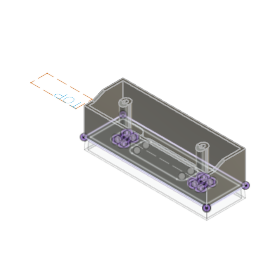
Eufy Doorbell Spacer (Autodesk Fusion 360 design; units mm, degrees)
Autodesk Fusion 360 part; units mm, degrees
note: some values were not read from the file. Chosen so that the rebuilt part matches the saved one: which pieces of a blend or face edit are solid.
sketch "Sketch1" plane through (0, 0, 0) normal (0, 0, 1) x (1, 0, 0) in component "Doorbell Back"
  line L0 (0, 0) -> (147, 0)
  line L1 (147, 0) -> (147, 45.8)
  line L2 (147, 45.8) -> (0, 45.8)
  line L3 (0, 45.8) -> (0, 0)
  line L4 (145.7948, 3.1933) -> (145.7948, 0) construction
  line L5 (145.7948, 43.4933) -> (145.7948, 45.8) construction
  line L6 (147, 22.9) -> (0, 22.9) construction
  line L7 (27.9, 21.95) -> (27.9, 23.85)
  arc A0 (27.9, 23.85) -> (23.8, 23.85) centre (25.85, 23.85) ccw
  line L8 (23.8, 23.85) -> (23.8, 21.95)
  arc A1 (23.8, 21.95) -> (27.9, 21.95) centre (25.85, 21.95) ccw
  line L9 (25.85, 21.95) -> (25.85, 23.85) construction
  line L10 (121, 21.95) -> (121, 23.85)
  arc A2 (121, 23.85) -> (116.9, 23.85) centre (118.95, 23.85) ccw
  line L11 (116.9, 23.85) -> (116.9, 21.95)
  arc A3 (116.9, 21.95) -> (121, 21.95) centre (118.95, 21.95) ccw
  line L12 (118.95, 21.95) -> (118.95, 23.85) construction
  line L13 (22.4, 31.3) -> (29.3, 31.3)
  line L14 (32.3, 28.3) -> (32.3, 17.5)
  line L15 (29.3, 14.5) -> (22.4, 14.5)
  line L16 (19.4, 17.5) -> (19.4, 28.3)
  line L17 (19.4, 31.3) -> (32.3, 14.5) construction
  line L18 (32.3, 31.3) -> (19.4, 14.5) construction
  arc A4 (19.4, 17.5) -> (22.4, 14.5) centre (22.4, 17.5) ccw
  arc A5 (29.3, 14.5) -> (32.3, 17.5) centre (29.3, 17.5) ccw
  arc A6 (22.4, 31.3) -> (19.4, 28.3) centre (22.4, 28.3) ccw
  arc A7 (32.3, 28.3) -> (29.3, 31.3) centre (29.3, 28.3) ccw
  line L19 (25.85, 22.9) -> (118.95, 22.9) construction
  line L20 (115.5, 31.3) -> (122.4, 31.3)
  line L21 (125.4, 28.3) -> (125.4, 17.5)
  line L22 (122.4, 14.5) -> (115.5, 14.5)
  line L23 (112.5, 17.5) -> (112.5, 28.3)
  line L24 (112.5, 31.3) -> (125.4, 14.5) construction
  line L25 (125.4, 31.3) -> (112.5, 14.5) construction
  arc A8 (115.5, 31.3) -> (112.5, 28.3) centre (115.5, 28.3) ccw
  arc A9 (125.4, 28.3) -> (122.4, 31.3) centre (122.4, 28.3) ccw
  arc A10 (122.4, 14.5) -> (125.4, 17.5) centre (122.4, 17.5) ccw
  arc A11 (112.5, 17.5) -> (115.5, 14.5) centre (115.5, 17.5) ccw
  point P0 (25.85, 22.9)
  point P1 (118.95, 22.9)
  point P2 (25.85, 22.9)
  point P3 (118.95, 22.9)
  dimension "d1" = 45.8
  dimension "d5" = 147
  dimension "d6" = 4.1
  dimension "d7" = 6
  dimension "d10" = 16.8
  dimension "d11" = 12.9
  dimension "d12" = 3
  dimension "d14" = 93.1
  dimension "d15" = 28.05
  constraint horizontal L0
  constraint vertical L1
  constraint horizontal L2
  constraint vertical L3
  constraint coincident L0.start L3.end
  constraint coincident L0 L4.end
  constraint perpendicular L0 L4
  constraint coincident L2 L5.end
  constraint perpendicular L2 L5
  constraint midpoint L1 L6.start
  constraint midpoint L3 L6.end
  constraint tangent L7 A0
  constraint tangent A0 L8
  constraint parallel L7 L8
  constraint tangent L8 A1
  constraint tangent L7 A1
  constraint perpendicular L6 L9
  constraint coincident L6 P2
  constraint midpoint L9 P2
  constraint tangent L10 A2
  constraint tangent A2 L11
  constraint parallel L10 L11
  constraint tangent L11 A3
  constraint tangent L10 A3
  constraint perpendicular L6 L12
  constraint midpoint L12 P3
  constraint equal L7 L11
  constraint equal A0 A2
  constraint coincident L6 P3
  constraint horizontal L13
  constraint perpendicular L13 L14
  constraint parallel L13 L15
  constraint parallel L14 L16
  constraint coincident L17 P2
  constraint coincident L18 P2
  constraint coincident P2 P0
  constraint coincident L18.end L15
  constraint coincident L18.end L16
  constraint tangent L15 A4
  constraint tangent L16 A4
  constraint coincident L17.end L14
  constraint coincident L17.end L15
  constraint tangent L14 A5
  constraint tangent L15 A5
  constraint equal A4 A5
  constraint coincident L17.start L16
  constraint coincident L17.start L13
  constraint tangent L16 A6
  constraint tangent L13 A6
  constraint coincident L18.start L14
  constraint coincident L18.start L13
  constraint tangent L14 A7
  constraint tangent L13 A7
  constraint equal A6 A7
  constraint equal A4 A6
  constraint coincident P3 P1
  constraint horizontal L20
  constraint perpendicular L20 L21
  constraint parallel L20 L22
  constraint parallel L21 L23
  constraint coincident L24 P3
  constraint coincident L25 P3
  constraint coincident L24.start L23
  constraint coincident L24.start L20
  constraint tangent L23 A8
  constraint tangent L20 A8
  constraint coincident L25.start L21
  constraint coincident L25.start L20
  constraint tangent L21 A9
  constraint tangent L20 A9
  constraint equal A8 A9
  constraint coincident L24.end L21
  constraint coincident L24.end L22
  constraint tangent L21 A10
  constraint tangent L22 A10
  constraint equal A8 A10
  constraint coincident L25.end L22
  constraint coincident L25.end L23
  constraint tangent L22 A11
  constraint tangent L23 A11
  constraint equal L13 L20
  constraint equal L16 L23
  constraint equal A10 A11
  constraint equal A5 A11
  measures "d1" distance of L0.end L1.end
  measures "d5" distance of L0.start L0.end
  measures "d6" distance of L10 L11
  measures "d10" distance of L18.start L17.end
  measures "d11" distance of L17.end L18.end
  measures "d12" radius of A4
  measures "d14" distance of P2 P3
  measures "d15" distance of L1 P3
extrude "Extrude1" add sketch "Sketch1" against normal blind 13.45 draft 3 contours L0 L1 L2 L3 | L13 L14 L15 L16 A4 A5 A6 A7 | L20 L21 L22 L23 A8 A9 A10 A11 makes body 1 in component "Doorbell Back"
extrude "Extrude2" add sketch "Sketch1" along normal blind 2.8 contours L13 L14 L15 L16 A4 A5 A6 A7 | L20 L21 L22 L23 A8 A9 A10 A11 bodies 1 in component "Doorbell Back"
fillet "Fillet1" radius 2 2 edges at (73.5, 45.8, 0) (73.5, 0, 0) on bodies 1 in component "Doorbell Back"
shell "Shell1" thickness 2.4 removed faces 9 at (27.665, 22.5833, -4.4833) at (24.1601, 24.0114, -6.725) at (24.2699, 23.2167, -8.9667) at (24.1601, 21.7886, -6.725) at (120.5301, 22.5833, -8.9667) at (117.2601, 24.0114, -6.725) at (138.5683, 22.5833, -13.45) at (117.135, 23.2167, -4.4833) at (120.6399, 21.7886, -6.725) on bodies 1 in component "Doorbell Back"
sketch "Sketch1 (2)" plane through (0, 0, 0) normal (0, 0, 1) x (-1, 0, 0) in component "Spacer"
  line L0 (-115.5, -31.3) -> (-122.4, -31.3)
  arc A0 (-125.4, -28.3) -> (-122.4, -31.3) centre (-122.4, -28.3) ccw
  line L1 (-125.4, -28.3) -> (-125.4, -17.5)
  arc A1 (-122.4, -14.5) -> (-125.4, -17.5) centre (-122.4, -17.5) ccw construction
  line L2 (-122.4, -14.5) -> (-115.5, -14.5) construction
  arc A2 (-112.5, -17.5) -> (-115.5, -14.5) centre (-115.5, -17.5) ccw construction
  line L3 (-112.5, -17.5) -> (-112.5, -28.3) construction
  arc A3 (-115.5, -31.3) -> (-112.5, -28.3) centre (-115.5, -28.3) ccw construction
  line L4 (-29.3, -14.5) -> (-22.4, -14.5) construction
  arc A4 (-19.4, -17.5) -> (-22.4, -14.5) centre (-22.4, -17.5) ccw construction
  line L5 (-19.4, -17.5) -> (-19.4, -28.3) construction
  arc A5 (-22.4, -31.3) -> (-19.4, -28.3) centre (-22.4, -28.3) ccw construction
  line L6 (-22.4, -31.3) -> (-29.3, -31.3) construction
  arc A6 (-32.3, -28.3) -> (-29.3, -31.3) centre (-29.3, -28.3) ccw construction
  line L7 (-32.3, -28.3) -> (-32.3, -17.5) construction
  arc A7 (-29.3, -14.5) -> (-32.3, -17.5) centre (-29.3, -17.5) ccw construction
  line L8 (0, -1.8979) -> (-147, -1.8979)
  line L9 (-147, -1.8979) -> (-147, -43.9021)
  line L10 (-147, -43.9021) -> (0, -43.9021)
  line L11 (0, -43.9021) -> (0, -1.8979)
  arc A8 (-121, -23.85) -> (-116.9, -23.85) centre (-118.95, -23.85) ccw
  line L12 (-121, -23.85) -> (-121, -21.95)
  arc A9 (-27.9, -23.85) -> (-23.8, -23.85) centre (-25.85, -23.85) ccw construction
  line L13 (-27.9, -23.85) -> (-27.9, -21.95)
  arc A10 (-116.9, -21.95) -> (-121, -21.95) centre (-118.95, -21.95) ccw
  arc A11 (-23.8, -21.95) -> (-27.9, -21.95) centre (-25.85, -21.95) ccw construction
  line L14 (-23.8, -21.95) -> (-23.8, -23.85)
  line L15 (-116.9, -21.95) -> (-116.9, -23.85)
  line L16 (-147.7049, 0.7049) -> (-147.7049, -46.5049)
  line L17 (-147.7049, -46.5049) -> (0.7049, -46.5049)
  line L18 (0.7049, 0.7049) -> (-147.7049, 0.7049)
  line L19 (0.7049, -46.5049) -> (0.7049, 0.7049)
  line L20 (0.6049, -46.4049) -> (-147.6049, -46.4049)
  line L21 (-147.6049, -46.4049) -> (-147.6049, 0.6049)
  line L22 (-147.6049, 0.6049) -> (0.6049, 0.6049)
  line L23 (0.6049, 0.6049) -> (0.6049, -46.4049)
  arc A12 (-23.8, -21.95) -> (-27.9, -21.95) centre (-25.85, -21.95) ccw
  line L24 (-23.8, -21.95) -> (-23.8, -23.85) construction
  arc A13 (-27.9, -23.85) -> (-23.8, -23.85) centre (-25.85, -23.85) ccw
  line L25 (-27.9, -23.85) -> (-27.9, -21.95) construction
  arc A14 (-29.3, -14.5) -> (-32.3, -17.5) centre (-29.3, -17.5) ccw construction
  line L26 (-32.3, -17.5) -> (-32.3, -28.3) construction
  arc A15 (-32.3, -28.3) -> (-29.3, -31.3) centre (-29.3, -28.3) ccw construction
  line L27 (-29.3, -31.3) -> (-22.4, -31.3) construction
  arc A16 (-22.4, -31.3) -> (-19.4, -28.3) centre (-22.4, -28.3) ccw construction
  line L28 (-19.4, -28.3) -> (-19.4, -17.5) construction
  arc A17 (-19.4, -17.5) -> (-22.4, -14.5) centre (-22.4, -17.5) ccw construction
  line L29 (-22.4, -14.5) -> (-29.3, -14.5) construction
  arc A18 (-116.9, -21.95) -> (-121, -21.95) centre (-118.95, -21.95) ccw
  line L30 (-116.9, -21.95) -> (-116.9, -23.85)
  arc A19 (-121, -23.85) -> (-116.9, -23.85) centre (-118.95, -23.85) ccw
  line L31 (-121, -23.85) -> (-121, -21.95)
  arc A20 (-115.5, -31.3) -> (-112.5, -28.3) centre (-115.5, -28.3) ccw construction
  line L32 (-112.5, -28.3) -> (-112.5, -17.5) construction
  arc A21 (-112.5, -17.5) -> (-115.5, -14.5) centre (-115.5, -17.5) ccw construction
  line L33 (-115.5, -14.5) -> (-122.4, -14.5) construction
  arc A22 (-122.4, -14.5) -> (-125.4, -17.5) centre (-122.4, -17.5) ccw construction
  line L34 (-125.4, -17.5) -> (-125.4, -28.3) construction
  arc A23 (-125.4, -28.3) -> (-122.4, -31.3) centre (-122.4, -28.3) ccw construction
  line L35 (-122.4, -31.3) -> (-115.5, -31.3) construction
  line L36 (-112.5, -17.5) -> (-112.5, -28.3) construction
  line L37 (-143.6049, -3.3951) -> (-3.3951, -3.3951)
  line L38 (-3.3951, -3.3951) -> (-3.3951, -42.4049)
  line L39 (-3.3951, -42.4049) -> (-143.6049, -42.4049)
  line L40 (-143.6049, -42.4049) -> (-143.6049, -3.3951)
  arc A24 (-29.3, -11.5) -> (-35.3, -17.5) centre (-29.3, -17.5) ccw
  line L41 (-35.3, -28.3) -> (-35.3, -17.5)
  arc A25 (-35.3, -28.3) -> (-29.3, -34.3) centre (-29.3, -28.3) ccw
  line L42 (-22.4, -34.3) -> (-29.3, -34.3)
  arc A26 (-22.4, -34.3) -> (-16.4, -28.3) centre (-22.4, -28.3) ccw
  line L43 (-16.4, -17.5) -> (-16.4, -28.3)
  arc A27 (-16.4, -17.5) -> (-22.4, -11.5) centre (-22.4, -17.5) ccw
  line L44 (-29.3, -11.5) -> (-22.4, -11.5)
  arc A28 (-115.5, -34.3) -> (-109.5, -28.3) centre (-115.5, -28.3) ccw
  line L45 (-109.5, -17.5) -> (-109.5, -28.3)
  arc A29 (-109.5, -17.5) -> (-115.5, -11.5) centre (-115.5, -17.5) ccw
  line L46 (-122.4, -11.5) -> (-115.5, -11.5)
  arc A30 (-122.4, -11.5) -> (-128.4, -17.5) centre (-122.4, -17.5) ccw
  line L47 (-128.4, -28.3) -> (-128.4, -17.5)
  arc A31 (-128.4, -28.3) -> (-122.4, -34.3) centre (-122.4, -28.3) ccw
  line L48 (-115.5, -34.3) -> (-122.4, -34.3)
  line L49 (-109.5, -22.9) -> (-35.3, -22.9) construction
  line L50 (-99.5, -34.3) -> (-45.3, -34.3)
  line L51 (-39.3, -28.3) -> (-39.3, -17.5)
  line L52 (-45.3, -11.5) -> (-99.5, -11.5)
  line L53 (-105.5, -17.5) -> (-105.5, -28.3)
  arc A32 (-105.5, -28.3) -> (-99.5, -34.3) centre (-99.5, -28.3) ccw
  arc A33 (-45.3, -34.3) -> (-39.3, -28.3) centre (-45.3, -28.3) ccw
  arc A34 (-39.3, -17.5) -> (-45.3, -11.5) centre (-45.3, -17.5) ccw
  arc A35 (-99.5, -11.5) -> (-105.5, -17.5) centre (-99.5, -17.5) ccw
  line L54 (35.3371, -43.8995) -> (89.7566, -43.8995) construction
  line L55 (89.7566, -43.8995) -> (89.7566, -24.1317) construction
  line L56 (89.7566, -24.1317) -> (35.3371, -24.1317) construction
  line L57 (35.3371, -24.1317) -> (35.3371, -43.8995) construction
  dimension "d25" = 0.1
  dimension "d26" = 0.1
  dimension "d27" = 0.1
  dimension "d28" = 0.1
  dimension "d29" = 4
  dimension "d30" = -3
  dimension "d31" = -3
  dimension "d45" = 4
  dimension "d46" = 4
  dimension "d47" = 6
  dimension "d50" = 26.4549
  dimension "d51" = 28.6549
  dimension "d52" = 10
  constraint horizontal L20
  constraint vertical L21
  constraint horizontal L22
  constraint vertical L23
  constraint midpoint L45 L49.start
  constraint midpoint L41 L49.end
  constraint horizontal L50
  constraint vertical L51
  constraint horizontal L52
  constraint vertical L53
  constraint collinear L44 L52
  constraint collinear L48 L50
  constraint tangent L53 A32
  constraint tangent L50 A32
  constraint tangent L51 A33
  constraint tangent L50 A33
  constraint equal A32 A33
  constraint tangent L51 A34
  constraint tangent L52 A34
  constraint equal A32 A34
  constraint tangent L53 A35
  constraint tangent L52 A35
  constraint equal A32 A35
  measures "d25" distance of L16 L21
  measures "d26" distance of L19 L23
  measures "d27" distance of L17 L20
  measures "d28" distance of L18 L22
  measures "d45" distance of L45 L53
  measures "d46" distance of L41.start L51
  measures "d47" radius of A32
  measures "d50" distance of L23 A9.centre
  measures "d51" distance of A8.centre L21
extrude "Extrude1'" add sketch "Sketch1 (2)" along normal blind 38.55 separate body contours L8 L9 L10 L11 | L20 L21 L22 L23 | L37 L38 L39 L40 | A24 L41 A25 L42 A26 L43 A27 L44 | A28 L45 A29 L46 A30 L47 A31 L48 | L50 L51 L52 L53 A32 A33 A34 A35 makes body 2 in component "Spacer"
extrude "Extrude4" cut sketch "Sketch1 (2)" along normal blind 2.8 contours A24 L41 A25 L42 A26 L43 A27 L44 | A28 L45 A29 L46 A30 L47 A31 L48 bodies 2 in component "Spacer"
shell "Shell1'" thickness 3 removed faces 1 at (138.7366, 22.5833, 38.55) on bodies 2 in component "Spacer"
extrude "Extrude5" cut sketch "Sketch1 (2)" along normal blind 3 contours L50 L51 L52 L53 A32 A33 A34 A35 bodies 2 in component "Spacer"
sketch "Sketch2" plane through (-0.6049, 0, 0) normal (-1, 0, 0) x (0, -1, 0) in component "Spacer"
  line L0 (-46.4049, 0) -> (0.6049, 0)
  line L1 (0.6049, 0) -> (0.6049, 38.55)
  line L2 (0.6049, 38.55) -> (-46.4049, 38.55)
  line L3 (-46.4049, 38.55) -> (-46.4049, 0)
  line L4 (0.6049, 33.05) -> (-9.3951, 33.05)
  line L5 (-9.3951, 33.05) -> (-21.3951, 38.55)
  line L6 (-22.9, 38.55) -> (-22.9, 48.1731) construction
  dimension "d55" = 10
  dimension "d57" = 12
  dimension "d58" = 5.5
  constraint coincident L1 L4.start
  constraint perpendicular L1 L4
  constraint coincident L2 L5.end
  constraint midpoint L2 L6.start
  constraint perpendicular L2 L6
  measures "d55" distance of L4.start L4.end
  measures "d57" horizontal distance of L4.end L5.end
  measures "d58" distance of L2 L4
extrude "Extrude6" cut sketch "Sketch2" against normal through all contours L1 L2 L4 L5 bodies 2 in component "Spacer"
component "Doorbell Back" placed x (1, 0, 0) y (0, 1, 0) z (0, 0, 1) at (0, 0, 0)
component "Spacer" placed x (1, 0, 0) y (0, 1, 0) z (0, 0, 1) at (0, 0, 0)
equation "d26 = d25"
equation "d27 = d25"
equation "d28 = d25"
equation "d32 = 52 mm - 13.45 mm"
equation "d46 = d45"
equation "d53 = 'TOP'"
named bodies: "Doorbell Back"
